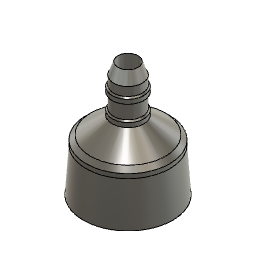
Pneumatic Connectors V1 - Blower V5 (Autodesk Fusion 360 design; units mm, degrees)
Autodesk Fusion 360 part; units mm, degrees
sketch "Sketch1" plane through (0, 0, 0) normal (0, 1, 0) x (1, 0, 0)
  circle A0 centre (0, 0) radius 15.5
  circle A1 centre (0, 0) radius 12.5
  dimension "d1" = 25
  dimension "d7" = 3
  constraint coincident A0.centre A1.centre
  measures "d1" diameter of A1
  measures "d7" distance of A0 A1
ref_plane "WorkPlane1" through (0, 15, 0) normal (0, 1, 0) x (0, 0, 1)
sketch "Sketch2" plane through (0, 15, 0) normal (0, 1, 0) x (1, 0, 0)
  circle A0 centre (0, 0) radius 11.5
  circle A1 centre (0, 0) radius 14.5
  dimension "d4" = 23
  dimension "d8" = 3
  constraint coincident A0.centre A1.centre
  measures "d4" diameter of A0
  measures "d8" distance of A0 A1
loft "Loft1" add profiles "Sketch1", "Sketch2" section 1 section 2
loft "Loft2" cut profiles "Sketch1", "Sketch2" section 1 contours A1 section 2 contours A0
extrude "Extrude3" add sketch "Sketch2" along normal blind 3 contours A0 | A1
sketch "Sketch3" plane through (0, 15, 0) normal (0, 1, 0) x (1, 0, 0)
  circle A0 centre (0, 0) radius 3
  circle A1 centre (0, 0) radius 5
  dimension "d9" = 6
  dimension "d10" = 2
  constraint coincident A0.centre A1.centre
  measures "d9" diameter of A0
  measures "d10" distance of A0 A1
extrude "Extrude1" add sketch "Sketch3" along normal blind 25
sketch "Sketch5" plane through (0, 40, 0) normal (0, 1, 0) x (-1, 0, 0)
  circle A0 centre (0, 0) radius 3
  circle A1 centre (0, 0) radius 5
  circle A2 centre (0, 0) radius 3.5
  constraint coincident A0.centre A1.centre
extrude "Extrude4" cut sketch "Sketch5" against normal up to surface (25 mm away) contours A0 | A2
chamfer "Chamfer1" distance 6 angle 45 1 edges at (-10.7218, 15, -4.1586)
chamfer "Chamfer2" distance 1.5 angle 45 1 edges at (-13.5187, 18, 5.2434)
ref_plane "WorkPlane2" through (0, 24, 0) normal (0, 1, 0) x (1, 0, 0)
sketch "Sketch6" plane through (0, 24, 0) normal (0, 1, 0) x (1, 0, 0)
  circle A0 centre (0, 0) radius 5.5
  circle A1 centre (0, 0) radius 3.5
  dimension "d22" = 11
  constraint coincident A0.centre A1.centre
  measures "d22" diameter of A0
extrude "Extrude5" add sketch "Sketch6" along normal blind 1.5
chamfer "Chamfer3" distance 0.5 angle 45 1 edges at (-4.6616, 25.5, 1.8081)
pattern_linear "R-Pattern1" count 2 spacing 7 along (0, 1, 0) of "Extrude5", "Chamfer3"
chamfer "Chamfer4" distance 1.5 distance2 4 1 edges at (-4.6616, 40, 1.8081) measured on face at (4.4684, 40, 0.4223)
chamfer "Chamfer5" distance 8 distance2 6 1 edges at (-4.6616, 18, -1.8081) measured on face at (10.2663, 18, 0.8943)
equation "d11 = 15 mm + 10 mm"
